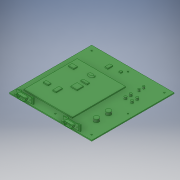
# Autodesk Inventor part: Board
Saved by Autodesk Inventor 2018 (Build 220112000, 112)
## iProperties
Created: 2021-04-09
Part Number: Board
Material: Generic
Document SubType Name: Modeling
Designer: Ramana Bharathi
Density: 0.5935 g/cm^3
Appearance: Smooth - Dark Forest Green
Mass: 50 g
Surface Area: 872.995 cm^2
Volume: 84.2461 cm^3
Author: Ramana Bharathi
Autodesk Inventor part; units mm, degrees
ref_plane "YZ Plane" through (0, 0, 0) normal (1, 0, 0) x (0, 1, 0)
sketch "Sketch1" plane through (0, 0, 0) normal (0, 1, 0) x (-1, 0, 0)
  line L0 (0, 0) -> (170, 0)
  line L1 (170, 0) -> (170, -170)
  line L2 (170, -170) -> (0, -170)
  line L3 (0, -170) -> (0, 0)
  dimension "d0" = 170
  dimension "d1" = 170
  constraints: 8 end point, 2 parallel, 1 horizontal, 1 perpendicular
  measures "d0" distance of L1.end L2.end
  measures "d1" distance of L0.end L1.end
extrude "Extrusion1" add sketch "Sketch1" along normal blind 2
sketch "Sketch2" plane through (0, 2, 0) normal (0, 1, 0) x (1, 0, 0)
  line L0 (-160, 10) -> (-10, 10)
  line L1 (-10, 10) -> (-10, 160)
  line L2 (-10, 160) -> (-160, 160)
  line L3 (-160, 160) -> (-160, 10)
  line L4 (-170, 170) -> (-170, 0) projected
  line L5 (0, 170) -> (-170, 170) projected
  circle A0 centre (-160, 10) radius 1.5
  circle A1 centre (-160, 85) radius 1.5
  circle A2 centre (-160, 160) radius 1.5
  circle A3 centre (-85, 10) radius 1.5
  circle A4 centre (-85, 85) radius 1.5
  circle A5 centre (-85, 160) radius 1.5
  circle A6 centre (-10, 10) radius 1.5
  circle A7 centre (-10, 85) radius 1.5
  circle A8 centre (-10, 160) radius 1.5
  point P0 (0, 0)
  dimension "d135" = 13
  dimension "d4" = 150
  dimension "d5" = 150
  dimension "d6" = 10
  dimension "d7" = 10
  dimension "d8" = 3
  dimension "d11" = 75
  dimension "d14" = 75
  constraints: 9 centre point, 8 end point, 2 horizontal, 2 parallel, 1 coincident, 1 perpendicular, 1 vertical, 16 other
  measures "d4" distance of L2.end L1.end
  measures "d5" distance of L1.end L0.end
  measures "d6" distance between parallel lines of L4 L3
  measures "d7" distance between parallel lines of L5 L2
  measures "d8" diameter of A0
  measures "d11" distance of A0.centre A1.centre
  measures "d14" distance of A0.centre A3.centre
sketch "Sketch3" plane through (0, 2, 0) normal (0, 1, 0) x (1, 0, 0)
  circle A0 centre (-140, 25) radius 2.5
  circle A1 centre (-70, 25) radius 2.5
  circle A2 centre (-140, 115) radius 2.5
  circle A3 centre (-70, 115) radius 2.5
  line L0 (-170, 170) -> (-170, 0) projected
  line L1 (-170, 0) -> (0, 0) projected
  dimension "d19" = 5
  dimension "d20" = 5
  dimension "d21" = 5
  dimension "d22" = 5
  dimension "d23" = 70
  dimension "d24" = 90
  dimension "d25" = 70
  dimension "d26" = 30
  dimension "d27" = 25
  dimension "d28" = 0
  dimension "d29" = 0
  dimension "d30" = 90
  constraints: 4 centre point
  measures "d19" diameter of A0
  measures "d20" diameter of A1
  measures "d21" diameter of A2
  measures "d22" diameter of A3
  measures "d23" distance of A1.centre A0.centre
  measures "d24" distance of A0.centre A2.centre
  measures "d25" distance of A3.centre A2.centre
  measures "d26" distance from line of L0 A0.centre
  measures "d27" distance from line of L1 A0.centre
  measures "d28" vertical distance of A1.centre A0.centre
  measures "d29" vertical distance of A3.centre A2.centre
  measures "d30" distance of A1.centre A3.centre
extrude "Extrusion3" add sketch "Sketch3" along normal blind 4
ref_plane "Work Plane1" through (0, 6, 0) normal (0, 1, 0) x (1, 0, 0)
sketch "Sketch5" plane through (0, 6, 0) normal (0, 1, 0) x (1, 0, 0)
  line L0 (-155, 125) -> (-55, 125) projected
  circle A0 centre (-140, 115) radius 2.5 projected
  circle A1 centre (-140, 25) radius 2.5 projected
  circle A2 centre (-70, 25) radius 2.5 projected
  circle A3 centre (-70, 115) radius 2.5 projected
  line L1 (-170, 0) -> (0, 0) projected
  line L2 (0, 0) -> (0, 170) projected
  line L3 (0, 170) -> (-170, 170) projected
  line L4 (-170, 170) -> (-170, 0) projected
  line L5 (-55, 125) -> (-55, 15) projected
  line L6 (-155, 15) -> (-155, 125) projected
  line L7 (-55, 15) -> (-155, 15) projected
extrude "Extrusion4" add sketch "Sketch5" along normal blind 2 contours L0 L5 L7 L6 | A0 | A1 | A2 | A3
sketch "Sketch6" plane through (0, 2, 0) normal (0, 1, 0) x (1, 0, 0)
  circle A0 centre (-29.6751, 64.4345) radius 5
  circle A1 centre (-29.6751, 39.5323) radius 5
  point P0 (0, 0)
  dimension "d40" = 10
  dimension "d41" = 10
  constraints: 2 centre point
  measures "d40" diameter of A0
  measures "d41" diameter of A1
extrude "Extrusion5" add sketch "Sketch6" along normal blind 6
sketch "Sketch7" plane through (0, 2, 0) normal (0, 1, 0) x (1, 0, 0)
  circle A0 centre (-39.0135, 108.8434) radius 2.5
  circle A1 centre (-39.0135, 119.7104) radius 2.5
  circle A2 centre (-25.561, 108.8434) radius 2.5
  circle A3 centre (-25.561, 119.7104) radius 2.5
  circle A4 centre (-39.0135, 136.7746) radius 2
  circle A5 centre (-39.0135, 146.4571) radius 2
  point P0 (0, 0)
  dimension "d44" = 5
  dimension "d45" = 5
  dimension "d46" = 5
  dimension "d47" = 5
  dimension "d48" = 4
  dimension "d49" = 4
  constraints: 6 centre point
  measures "d44" diameter of A0
  measures "d45" diameter of A1
  measures "d46" diameter of A2
  measures "d47" diameter of A3
  measures "d48" diameter of A4
  measures "d49" diameter of A5
extrude "Extrusion6" add sketch "Sketch7" along normal blind 4
sketch "Sketch8" plane through (0, 2, 0) normal (0, 1, 0) x (1, 0, 0)
  line L0 (-115.7953, 153.2524) -> (-109.7953, 153.2524)
  line L1 (-109.7953, 153.2524) -> (-109.7953, 143.2524)
  line L2 (-109.7953, 143.2524) -> (-115.7953, 143.2524)
  line L3 (-115.7953, 143.2524) -> (-115.7953, 153.2524)
  line L4 (-93.1036, 153.2524) -> (-89.1036, 153.2524)
  line L5 (-89.1036, 153.2524) -> (-89.1036, 149.2524)
  line L6 (-89.1036, 149.2524) -> (-93.1036, 149.2524)
  line L7 (-93.1036, 149.2524) -> (-93.1036, 153.2524)
  point P0 (0, 0)
  dimension "d52" = 6
  dimension "d53" = 10
  dimension "d54" = 4
  dimension "d55" = 4
  constraints: 16 end point, 4 parallel, 2 horizontal, 2 perpendicular, 1 point on line
  measures "d52" distance of L1.end L2.end
  measures "d53" distance of L0.end L1.end
  measures "d54" distance of L5.end L6.end
  measures "d55" distance of L4.end L5.end
extrude "Extrusion7" add sketch "Sketch8" along normal blind 2
ref_plane "Work Plane2" through (-155, 6, 0) normal (0, 0, 1) x (1, 0, 0)
sketch "Sketch9" plane through (-155, 6, 0) normal (0, 0, 1) x (1, 0, 0)
  line L0 (0, 0) -> (100, 0) projected
  line L1 (0, 0) -> (32, 0)
  line L2 (32, 0) -> (32, 11)
  line L3 (32, 11) -> (0, 11)
  line L4 (0, 11) -> (0, 0)
  line L5 (97, 0) -> (129, 0)
  line L6 (129, 0) -> (129, 11)
  line L7 (129, 11) -> (97, 11)
  line L8 (97, 11) -> (97, 0)
  point P0 (155, -6)
  dimension "d59" = 32
  dimension "d60" = 11
  dimension "d61" = 32
  dimension "d62" = 11
  dimension "d63" = 65
  constraints: 16 end point, 4 parallel, 2 horizontal, 2 perpendicular, 1 point on line
  measures "d59" distance of L3.end L2.end
  measures "d60" distance of L2.end L1.end
  measures "d61" distance of L7.end L6.end
  measures "d62" distance of L6.end L5.end
  measures "d63" distance between parallel lines of L2 L8
extrude "Extrusion8" add sketch "Sketch9" along normal blind 1
sketch "Sketch10" plane through (-155, 6, 1) normal (0, 0, 1) x (1, 0, 0)
  circle A0 centre (3.5, 5.5) radius 1.25
  circle A1 centre (28.5, 5.5) radius 1.25
  line L0 (0, 0) -> (32, 0) projected
  line L1 (0, 11) -> (0, 0) projected
  line L2 (8.3056, 9) -> (23.6946, 9)
  line L3 (22.3465, 2) -> (9.6549, 2)
  line L4 (32, 11) -> (0, 11) projected
  line L5 (7.3402, 7.7395) -> (8.6894, 2.7395)
  line L6 (0, 2) -> (100, 2) projected
  line L7 (24.6602, 7.7397) -> (23.312, 2.7397)
  arc A2 (24.6602, 7.7397) -> (23.6946, 9) centre (23.6946, 8) ccw
  arc A3 (22.3465, 2) -> (23.312, 2.7397) centre (22.3465, 3) ccw
  arc A4 (8.6894, 2.7395) -> (9.6549, 2) centre (9.6549, 3) ccw
  arc A5 (8.3056, 9) -> (7.3402, 7.7395) centre (8.3056, 8) ccw
  circle A6 centre (9.6549, 6.667) radius 0.25
  circle A7 centre (9.6549, 4.334) radius 0.25
  circle A8 centre (11.4049, 6.667) radius 0.25
  circle A9 centre (11.4049, 4.334) radius 0.25
  circle A10 centre (13.1549, 6.667) radius 0.25
  circle A11 centre (13.1549, 4.334) radius 0.25
  circle A12 centre (14.9049, 6.667) radius 0.25
  circle A13 centre (14.9049, 4.334) radius 0.25
  circle A14 centre (16.6549, 6.667) radius 0.25
  circle A15 centre (16.6549, 4.334) radius 0.25
  circle A16 centre (18.4049, 6.667) radius 0.25
  circle A17 centre (18.4049, 4.334) radius 0.25
  circle A18 centre (20.1549, 6.667) radius 0.25
  circle A19 centre (20.1549, 4.334) radius 0.25
  circle A20 centre (21.9049, 6.667) radius 0.25
  circle A21 centre (21.9049, 4.334) radius 0.25
  line L8 (23.6946, 9.4) -> (8.3056, 9.4)
  arc A22 (8.3056, 9.4) -> (6.954, 7.6353) centre (8.3056, 8) ccw
  line L9 (6.954, 7.6353) -> (8.3032, 2.6353)
  arc A23 (8.3032, 2.6353) -> (9.6549, 1.6) centre (9.6549, 3) ccw
  line L10 (9.6549, 1.6) -> (22.3465, 1.6)
  arc A24 (22.3465, 1.6) -> (23.6982, 2.6355) centre (22.3465, 3) ccw
  line L11 (23.6982, 2.6355) -> (25.0464, 7.6355)
  arc A25 (25.0464, 7.6355) -> (23.6946, 9.4) centre (23.6946, 8) ccw
  circle A26 centre (100.5, 5.5) radius 1.25
  circle A27 centre (125.5, 5.5) radius 1.25
  line L12 (105.3031, 9) -> (120.6922, 9)
  line L13 (119.344, 2) -> (106.6524, 2)
  line L14 (104.3377, 7.7395) -> (105.6869, 2.7395)
  line L15 (121.6577, 7.7397) -> (120.3095, 2.7397)
  arc A28 (121.6577, 7.7397) -> (120.6922, 9) centre (120.6922, 8) ccw
  arc A29 (119.344, 2) -> (120.3095, 2.7397) centre (119.344, 3) ccw
  arc A30 (105.6869, 2.7395) -> (106.6524, 2) centre (106.6524, 3) ccw
  arc A31 (105.3031, 9) -> (104.3377, 7.7395) centre (105.3031, 8) ccw
  circle A32 centre (106.6524, 6.667) radius 0.25
  circle A33 centre (106.6524, 4.334) radius 0.25
  circle A34 centre (108.4024, 6.667) radius 0.25
  circle A35 centre (108.4024, 4.334) radius 0.25
  circle A36 centre (110.1524, 6.667) radius 0.25
  circle A37 centre (110.1524, 4.334) radius 0.25
  circle A38 centre (111.9024, 6.667) radius 0.25
  circle A39 centre (111.9024, 4.334) radius 0.25
  circle A40 centre (113.6524, 6.667) radius 0.25
  circle A41 centre (113.6524, 4.334) radius 0.25
  circle A42 centre (115.4024, 6.667) radius 0.25
  circle A43 centre (115.4024, 4.334) radius 0.25
  circle A44 centre (117.1524, 6.667) radius 0.25
  circle A45 centre (117.1524, 4.334) radius 0.25
  circle A46 centre (118.9024, 6.667) radius 0.25
  circle A47 centre (118.9024, 4.334) radius 0.25
  line L16 (120.6922, 9.4) -> (105.3031, 9.4)
  arc A48 (105.3031, 9.4) -> (103.9515, 7.6353) centre (105.3031, 8) ccw
  line L17 (103.9515, 7.6353) -> (105.3007, 2.6353)
  arc A49 (105.3007, 2.6353) -> (106.6524, 1.6) centre (106.6524, 3) ccw
  line L18 (106.6524, 1.6) -> (119.344, 1.6)
  arc A50 (119.344, 1.6) -> (120.6957, 2.6355) centre (119.344, 3) ccw
  line L19 (120.6957, 2.6355) -> (122.0439, 7.6355)
  arc A51 (122.0439, 7.6355) -> (120.6922, 9.4) centre (120.6922, 8) ccw
  line L20 (97, 11) -> (97, 0) projected
  line L21 (97, 0) -> (129, 0) projected
  point P0 (155, -6)
  point P1 (8.8889, 2)
  point P2 (23.1125, 2)
  point P3 (105.8865, 2)
  point P4 (120.1101, 2)
  dimension "d66" = 2.5
  dimension "d67" = 2.5
  dimension "d68" = 25
  dimension "d69" = 5.5
  dimension "d70" = 5.5
  dimension "d71" = 3.5
  dimension "d74" = 2
  dimension "d78" = 1
  dimension "d79" = 0.5
  dimension "d80" = 2.333
  dimension "d83" = 2.333
  dimension "d86" = 1.75
  dimension "d89" = 0.4
  dimension "d94" = 2.5
  dimension "d95" = 2.5
  dimension "d96" = 25
  dimension "d97" = 1
  dimension "d98" = 0.5
  dimension "d99" = 2.333
  dimension "d100" = 2.333
  dimension "d101" = 1.75
  dimension "d102" = 0.4
  dimension "d103" = 3.5
  dimension "d104" = 5.5
  dimension "d105" = 5.5
  constraints: 52 centre point, 32 end point, 32 point on circle, 16 tangent, 7 point on line, 6 equal radius, 4 parallel, 3 horizontal, 1 vertical, 48 other
  measures "d66" diameter of A0
  measures "d67" diameter of A1
  measures "d68" distance of A1.centre A0.centre
  measures "d69" distance from line of L0 A0.centre
  measures "d70" distance from line of L0 A1.centre
  measures "d71" distance from line of L1 A0.centre
  measures "d74" distance between parallel lines of L4 L2
  measures "d78" radius of A2
  measures "d79" diameter of A6
  measures "d80" distance from line of A6.centre L2
  measures "d83" distance of A6.centre A7.centre
  measures "d86" distance of A6.centre A8.centre
  measures "d89" distance between parallel lines of L2 L8
  measures "d94" diameter of A26
  measures "d95" diameter of A27
  measures "d96" distance of A27.centre A26.centre
  measures "d97" radius of A28
  measures "d98" diameter of A32
  measures "d99" distance from line of A32.centre L12
  measures "d100" distance of A32.centre A33.centre
  measures "d101" distance of A32.centre A34.centre
  measures "d102" distance between parallel lines of L12 L16
  measures "d103" distance from line of L20 A26.centre
  measures "d104" distance from line of L21 A26.centre
  measures "d105" distance from line of L21 A27.centre
extrude "Extrusion9" add sketch "Sketch10" along normal blind 6 contours A0 | A1 | A5 L5 A4 L6 A23 L9 A22 L8 A25 L11 A24 A3 L7 A2 L2 | L3 L6 A24 L10 A23 | A6 | A7 | A8 | A9 | A10 | A11 | A12 | A13 | A14 | A15 | A16 | A17 | A18 | A19 | A20 | A21 | A26 | A27 | A32 | A33 | A34 | A35 | A36 | A37 | A38 | A39 | A40 | A41 | A42 | A43 | A44 | A45 | A46 | A47 | A51 L19 A50 L18 A49 L17 A48 L16
sketch "Sketch11" plane through (-155, 6, 1) normal (0, 0, 1) x (1, 0, 0)
  circle A0 centre (3.5, 5.5) radius 1.25 projected
  circle A1 centre (28.5, 5.5) radius 1.25 projected
  circle A2 centre (100.5, 5.5) radius 1.25 projected
  circle A3 centre (125.5, 5.5) radius 1.25 projected
  point P0 (155, -6)
extrude "Extrusion10" add sketch "Sketch11" against normal blind 4
sketch "Sketch14" plane through (-29.5, 11.5, -3) normal (0, 0, -1) x (-1, 0, 0)
  circle A0 centre (0, 0) radius 1.25 projected
  circle A1 centre (25, 0) radius 1.25 projected
  circle A2 centre (97, 0) radius 1.25 projected
  circle A3 centre (122, 0) radius 1.25 projected
  line L0 (-2.5, 2.5) -> (2.5, 2.5)
  line L1 (2.5, 2.5) -> (2.5, -2.5)
  line L2 (2.5, -2.5) -> (-2.5, -2.5)
  line L3 (-2.5, -2.5) -> (-2.5, 2.5)
  line L4 (22.5, 2.5) -> (27.5, 2.5)
  line L5 (27.5, 2.5) -> (27.5, -2.5)
  line L6 (27.5, -2.5) -> (22.5, -2.5)
  line L7 (22.5, -2.5) -> (22.5, 2.5)
  line L8 (94.5, 2.5) -> (99.5, 2.5)
  line L9 (99.5, 2.5) -> (99.5, -2.5)
  line L10 (99.5, -2.5) -> (94.5, -2.5)
  line L11 (94.5, -2.5) -> (94.5, 2.5)
  line L12 (119.5, 2.5) -> (124.5, 2.5)
  line L13 (124.5, 2.5) -> (124.5, -2.5)
  line L14 (124.5, -2.5) -> (119.5, -2.5)
  line L15 (119.5, -2.5) -> (119.5, 2.5)
  point P0 (-29.5, -11.5)
  dimension "d112" = 5
  dimension "d113" = 5
  dimension "d114" = 2.5
  dimension "d115" = 2.5
  dimension "d116" = 5
  dimension "d117" = 5
  dimension "d118" = 5
  dimension "d119" = 5
  dimension "d120" = 5
  dimension "d121" = 5
  dimension "d122" = 2.5
  dimension "d123" = 2.5
  dimension "d124" = 2.5
  dimension "d125" = 2.5
  dimension "d126" = 2.5
  dimension "d127" = 2.5
  constraints: 32 end point, 8 parallel, 4 horizontal, 4 perpendicular
  measures "d112" distance of L1.end L2.end
  measures "d113" distance of L0.end L1.end
  measures "d114" distance from line of A0.centre L0
  measures "d115" distance from line of A0.centre L3
  measures "d116" distance of L5.end L6.end
  measures "d117" distance of L4.end L5.end
  measures "d118" distance of L9.end L10.end
  measures "d119" distance of L8.end L9.end
  measures "d120" distance of L13.end L14.end
  measures "d121" distance of L12.end L13.end
  measures "d122" distance from line of A3.centre L12
  measures "d123" distance from line of A3.centre L15
  measures "d124" distance from line of A2.centre L8
  measures "d125" distance from line of L11 A2.centre
  measures "d126" distance from line of A1.centre L4
  measures "d127" distance from line of A1.centre L7
extrude "Extrusion12" add sketch "Sketch14" along normal blind 2 contours A0 | A1 | A2 | A3 | L0 L1 L2 L3 | L4 L5 L6 L7 | L8 L9 L10 L11 | L12 L13 L14 L15
sketch "Sketch15" plane through (-154, 14, -3) normal (0, 1, 0) x (1, 0, 0)
  line L0 (5, 0) -> (0, 0) projected
  line L1 (5, 0) -> (5, 2) projected
  line L2 (0, 2) -> (5, 2) projected
  line L3 (0, 0) -> (0, 2) projected
  line L4 (30, 0) -> (25, 0) projected
  line L5 (30, 0) -> (30, 2) projected
  line L6 (25, 2) -> (30, 2) projected
  line L7 (25, 0) -> (25, 2) projected
  line L8 (102, 0) -> (97, 0) projected
  line L9 (102, 0) -> (102, 2) projected
  line L10 (97, 2) -> (102, 2) projected
  line L11 (97, 0) -> (97, 2) projected
  line L12 (127, 0) -> (122, 0) projected
  line L13 (127, 0) -> (127, 2) projected
  line L14 (122, 2) -> (127, 2) projected
  line L15 (122, 0) -> (122, 2) projected
  point P0 (154, -3)
extrude "Extrusion13" add sketch "Sketch15" against normal up to surface (12 mm away)
sketch "Sketch16" plane through (0, 8, 0) normal (0, 1, 0) x (1, 0, 0)
  line L0 (-145.913, 51.9259) -> (-135.913, 51.9259)
  line L1 (-135.913, 51.9259) -> (-135.913, 45.9259)
  line L2 (-135.913, 45.9259) -> (-145.913, 45.9259)
  line L3 (-145.913, 45.9259) -> (-145.913, 51.9259)
  line L4 (-110.2612, 80.1273) -> (-97.2612, 80.1273)
  line L5 (-97.2612, 80.1273) -> (-97.2612, 67.1273)
  line L6 (-97.2612, 67.1273) -> (-110.2612, 67.1273)
  line L7 (-110.2612, 67.1273) -> (-110.2612, 80.1273)
  line L8 (-110.2612, 92.5936) -> (-97.2612, 92.5936)
  line L9 (-97.2612, 92.5936) -> (-97.2612, 87.5936)
  line L10 (-97.2612, 87.5936) -> (-110.2612, 87.5936)
  line L11 (-110.2612, 87.5936) -> (-110.2612, 92.5936)
  line L12 (-149.4901, 109.2917) -> (-138.4901, 109.2917)
  line L13 (-138.4901, 109.2917) -> (-138.4901, 101.2917)
  line L14 (-138.4901, 101.2917) -> (-149.4901, 101.2917)
  line L15 (-149.4901, 101.2917) -> (-149.4901, 109.2917)
  line L16 (-122.1557, 54.7371) -> (-115.1557, 54.7371)
  line L17 (-115.1557, 54.7371) -> (-115.1557, 41.7371)
  line L18 (-115.1557, 41.7371) -> (-122.1557, 41.7371)
  line L19 (-122.1557, 41.7371) -> (-122.1557, 54.7371)
  ellipse E0 centre (-110.2612, 109.2917) end of major axis (-103.1081, 109.2917) minor radius 4.7827
  point P0 (0, 0)
  dimension "d132" = 10
  dimension "d133" = 6
  dimension "d134" = 13
  dimension "d135" = 13
  dimension "d136" = 5
  dimension "d137" = 11
  dimension "d138" = 8
  dimension "d139" = 7
  dimension "d140" = 13
  constraints: 40 end point, 10 parallel, 5 horizontal, 5 perpendicular, 2 point on line, 2 other
  measures "d132" distance of L1.end L2.end
  measures "d133" distance of L0.end L1.end
  measures "d134" distance of L5.end L6.end
  measures "d135" distance of L4.end L5.end
  measures "d136" distance of L8.end L9.end
  measures "d137" distance of L13.end L14.end
  measures "d138" distance of L12.end L13.end
  measures "d139" distance of L17.end L18.end
  measures "d140" distance of L16.end L17.end
extrude "Extrusion14" add sketch "Sketch16" along normal blind 2
fillet "Fillet1" radius 2 1 edges at (-117.4142, 10, -109.2917)
hole "Hole1" at (-160, 2, -10) at (-160, 2, -85) at (-160, 2, -160) at (-85, 2, -10) at (-85, 2, -160) at (-10, 2, -10) at (-10, 2, -85) at (-10, 2, -160) at (-85, 2, -85) direction (0, -1, 0) diameter 3 end through all
body "Solid1"
